Autodesk Inventor part; units mm, degrees
(part 2 of 2)
sketch "草图7" plane through (0, 227, 0) normal (0, 1, 0) x (-1, 0, 0)
  line L0 (-24, 30.5) -> (24, 30.5)
  line L1 (24, 30.5) -> (24, 42.5)
  line L2 (24, 42.5) -> (-24, 42.5)
  line L3 (-24, 42.5) -> (-24, 30.5)
  line L4 (-5, 10) -> (5, 10)
  line L5 (5, 10) -> (5, 63)
  line L6 (5, 63) -> (-5, 63)
  line L7 (-5, 63) -> (-5, 10)
  line L8 (-77.0684, 73) -> (-71.0647, 73) projected
  line L9 (-71.0647, 73) -> (-71.0647, 0) projected
  line L10 (-71.0647, 0) -> (-77.0684, 0) projected
  line L11 (-77.0684, 0) -> (-77.0684, 73) projected
  line L12 (-65.2267, 73) -> (-56.8486, 73) projected
  line L13 (-56.8486, 73) -> (-56.8486, 0) projected
  line L14 (-56.8486, 0) -> (-65.2267, 0) projected
  line L15 (-65.2267, 0) -> (-65.2267, 73) projected
  line L16 (-53.3398, 73) -> (53.3398, 73) projected
  line L17 (53.3398, 73) -> (53.3398, 0) projected
  line L18 (53.3398, 0) -> (-53.3398, 0) projected
  line L19 (-53.3398, 0) -> (-53.3398, 73) projected
  line L20 (56.8486, 73) -> (65.2267, 73) projected
  line L21 (65.2267, 73) -> (65.2267, 0) projected
  line L22 (65.2267, 0) -> (56.8486, 0) projected
  line L23 (56.8486, 0) -> (56.8486, 73) projected
  line L24 (71.0647, 73) -> (77.0684, 73) projected
  line L25 (77.0684, 73) -> (77.0684, 0) projected
  line L26 (77.0684, 0) -> (71.0647, 0) projected
  line L27 (71.0647, 0) -> (71.0647, 73) projected
  line L28 (0, -26.5) -> (0, 99.5) projected
  line L29 (226, 0) -> (-226, 0) projected
  line L30 (-226, 73) -> (226, 73) projected
  line L31 (-198.992, 36.5) -> (190.1782, 36.5)
  point P0 (0, 0)
  dimension "d78" = 12
  dimension "d79" = 48
  dimension "d80" = 10
  dimension "d81" = 53
  dimension "d82" = 36.5
  constraints: 18 end point, 4 parallel, 3 horizontal, 2 perpendicular, 6 other
  measures "d78" distance of L2.end L0.start
  measures "d79" distance of L0.start L0.end
  measures "d80" distance of L4.start L4.end
  measures "d81" distance of L4.end L5.end
  measures "d82" distance of the line from the sketch origin of L31
loft "放样1" add profiles "草图5", "草图7" contours all / L3 L31 L7 L0 | L7 L31 L28 L0 | L0 L28 L4 L7 | L3 L2 L7 L31 | L28 L31 L5 L0 | L0 L5 L4 L28 | L7 L2 L28 L31 | L5 L31 L1 L0 | L28 L2 L5 L31 | L7 L6 L28 L2 | L5 L2 L1 L31 | L28 L6 L5 L2
extrude "拉伸5" add sketch "草图5" against normal blind 10 separate body contours L4 L1 L6 L3 | L3 L6 L5 L4 | L4 L7 L6 L1
combine bodies "合并1" operation type add bodies to combine 1 2
pattern_circular "环形阵列1" count 6 over 360 about axis through (0, 0, 0) along (0, 0, 1) of "放样1", "合并1" bodies 1
sketch "草图8" plane through (-49.2808, 34.2258, 30.5) normal (0, 0, -1) x (-0.8660254, 0.5, 0)
  line L0 (-56.2721, 61.0955) -> (31.71, 201.6483) projected
  circle A0 centre (-59.7913, -5) radius 226 projected
  line L1 (-63.3105, 61.0955) -> (-151.2926, 201.6483) projected
  line L2 (-56.2721, 61.0955) -> (-59.7913, 55) projected
  line L3 (-63.3105, 61.0955) -> (-59.7913, 55) projected
  point P0 (-168.4335, 193.1738)
  point P1 (48.8509, 193.1738)
extrude "拉伸10" add sketch "草图8" against normal up to surface (12 mm away) contours L2 L3 L1 A0 L0 picked at (-115.4629, 157.3233) bodies 1
sketch "草图9" plane through (5, 59.7913, 30.5) normal (0, 0, -1) x (-1, 0, 0)
  circle A0 centre (5, -59.7913) radius 214
  circle A1 centre (5, -59.7913) radius 72
  line L0 (-25, -0.7913) -> (-19.0817, 164.922) projected
  line L1 (-31.0955, -4.3105) -> (-177.5666, 73.4207) projected
  line L2 (-25, -0.7913) -> (-25, -7.8298) projected
  line L3 (-31.0955, -4.3105) -> (-25, -7.8298) projected
  arc A2 (-20.8842, 114.4522) -> (-59.9735, 144.1068) centre (-50.865, 115.523) ccw
  arc A3 (-139.0942, 98.4264) -> (-132.9572, 49.7468) centre (-118.8941, 76.2464) ccw
  arc A4 (-27.4043, 4.5046) -> (-24.6578, 8.7911) centre (-29.6546, 8.9696) ccw
  arc A5 (-39.5652, 0.1843) -> (-34.4797, 0.4196) centre (-37.2214, 4.6009) ccw
  point P0 (5, -59.7913)
  dimension "d109" = 428
  dimension "d110" = 144
  dimension "d111" = 60
  dimension "d112" = 60
  dimension "d114" = 10
  dimension "d115" = 10
  constraints: 12 point on circle, 8 tangent, 6 centre point, 4 point on line, 2 coincident
  measures "d109" diameter of A0
  measures "d110" diameter of A1
  measures "d111" diameter of A2
  measures "d112" diameter of A3
  measures "d114" diameter of A4
  measures "d115" diameter of A5
extrude "拉伸11" cut sketch "草图9" against normal up to surface (12 mm away) contours A2 L0 A4 A1 A5 L1 A3 A0 bodies 1
pattern_circular "环形阵列3" count 6 over 360 about axis through (0, 0, 0) along (0, 0, 1) of "拉伸11", "拉伸10" bodies 1
equation "\"d0\" = da_da"
equation "\"d1\" = da_b"
equation "\"d3\" = da_dw"
equation "\"d114\" = d115"
equation "\"d16\" = da_aw"
equation "\"d43\" = da_aw"
equation "\"d46\" = da_aw"
equation "\"da_da\" = 484"
equation "\"da_b\" = 73"
equation "\"da_dw\" = 476"
equation "\"da_aw\" = 276"
body "Solid1"
body "Srf1"
